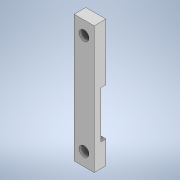
# Autodesk Inventor part: gps_cable_holder
Saved by Autodesk Inventor 2021 (Build 250183000, 183)
## iProperties
Created: 2020-12-14
Part Number: gps_cable_holder
Material: Generic
Document SubType Name: Modeling
Designer: Mateusz
Density: 1 g/cm^3
Appearance: Default
Author: Mateusz
Autodesk Inventor part; units mm, degrees
ref_plane "YZ Plane" through (0, 0, 0) normal (1, 0, 0) x (0, 1, 0)
ref_plane "XZ Plane" through (0, 0, 0) normal (0, 1, 0) x (-1, 0, 0)
ref_plane "Work Plane1" through (0, 0, 0) normal (0, 0, 1) x (1, 0, 0)
sketch "Sketch1" plane through (0, 0, 0) normal (0, 0, 1) x (1, 0, 0)
  circle A0 centre (26.8, 19.857) radius 1.45 projected
  circle A1 centre (26.8001, -10.143) radius 1.4501 projected
  line L0 (26.8, 23.857) -> (24.8, 23.857)
  line L1 (24.8, 23.857) -> (23.8, 23.857)
  line L2 (23.8, 23.857) -> (23.8, -10.143)
  line L3 (23.8, -10.143) -> (23.8, -14.143)
  line L4 (23.8, -14.143) -> (26.8, -14.143)
  line L5 (26.8, -14.143) -> (29.8, -14.143)
  line L6 (29.8, -14.143) -> (29.8, 23.857)
  line L7 (29.8, 23.857) -> (26.8, 23.857)
  line L8 (26.8, 6.857) -> (29.8, 6.857)
  line L9 (26.8, 6.857) -> (23.8, 6.857)
  line L10 (26.8, -7.143) -> (23.8, -7.143)
  line L11 (26.8, -7.143) -> (29.8, -7.143)
  point P0 (0, 0)
  dimension "d0" = 4
  dimension "d1" = 2
  dimension "d2" = 1
  dimension "d3" = 4
  dimension "d4" = 3
  dimension "d6" = 3
  constraints: 24 end point, 8 point on line, 6 perpendicular, 1 midpoint
  measures "d0" distance of A0.centre L0.start
  measures "d1" distance of L0.start L0.end
  measures "d2" distance of L0.end L1.end
  measures "d3" distance of L2.end L3.end
  measures "d4" distance of L4.end L5.end
  measures "d6" distance of A1.centre L10.start
extrude "Extrusion1" add sketch "Sketch1" along normal blind 1.5 contours L7 L6 L8 L9 L2 L1 L0 | L6 L5 L4 L3 L2 L10 L11
sketch "Sketch2" plane through (0, 0, 1.5) normal (0, 0, 1) x (1, 0, 0)
  line L0 (23.8, 23.857) -> (23.8, 6.857) projected
  line L1 (23.8, 6.857) -> (29.8, 6.857) projected
  line L2 (29.8, 6.857) -> (29.8, 23.857) projected
  line L3 (29.8, 23.857) -> (23.8, 23.857) projected
  circle A0 centre (26.8, 19.857) radius 1.45 projected
  line L4 (23.8, 23.857) -> (23.8, -10.143) projected
  line L5 (29.8, -14.143) -> (29.8, 23.857) projected
  line L6 (29.8, -14.143) -> (29.8, -7.143) projected
  line L7 (29.8, -7.143) -> (23.8, -7.143) projected
  line L8 (23.8, -7.143) -> (23.8, -14.143) projected
  line L9 (23.8, -14.143) -> (29.8, -14.143) projected
  circle A1 centre (26.8001, -10.143) radius 1.4501 projected
  point P0 (0, 0)
extrude "Extrusion2" add sketch "Sketch2" along normal blind 2
body "Solid1"
